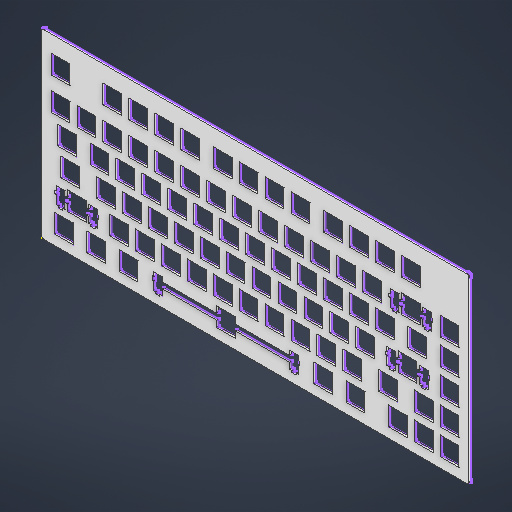
# Autodesk Inventor part: Keyboard_Plate
Saved by Autodesk Inventor 2026.1 (Build 301233000, 233)
## iProperties
Created: 2025-11-09
Part Number: Keyboard_Plate
Material: Generic
Document SubType Name: Modeling
Designer: avani
Density: 1 g/cm^3
Appearance: Default
Autodesk Inventor part; units mm, degrees
ref_plane "YZ Plane" through (0, 0, 0) normal (1, 0, 0) x (0, 1, 0)
ref_plane "XZ Plane" through (0, 0, 0) normal (0, 1, 0) x (-1, 0, 0)
ref_plane "XY Plane" through (0, 0, 0) normal (0, 0, 1) x (1, 0, 0)
sketch "Sketch1" plane through (0, 0, 0) normal (0, 0, 1) x (1, 0, 0)
  point P0 (0, 0)
sketch3d "3D 0"
sketch "Sketch2" plane through (0, 0, 0) normal (0, 0, 1) x (1, 0, 0)
  line L0 (2.096, 0.2549) -> (1.9389, 0.2604) projected
  line L1 (1.9389, 0.2604) -> (1.7818, 0.2797) projected
  line L2 (1.7818, 0.2797) -> (1.6288, 0.3087) projected
  line L3 (0.9192, 0.6367) -> (0.7965, 0.7331) projected
  line L4 (1.0501, 0.5498) -> (0.9192, 0.6367) projected
  line L5 (1.1879, 0.4727) -> (1.0501, 0.5498) projected
  line L6 (1.3298, 0.4065) -> (1.1879, 0.4727) projected
  line L7 (1.4759, 0.3528) -> (1.3298, 0.4065) projected
  line L8 (1.6288, 0.3087) -> (1.4759, 0.3528) projected
  line L9 (0.6808, 0.8406) -> (0.5746, 0.955) projected
  line L10 (0.5746, 0.955) -> (0.4768, 1.0776) projected
  line L11 (0.4768, 1.0776) -> (0.39, 1.2099) projected
  line L12 (0.39, 1.2099) -> (0.3128, 1.3463) projected
  line L13 (0.3128, 1.3463) -> (0.248, 1.4897) projected
  line L14 (0.7965, 0.7331) -> (0.6808, 0.8406) projected
  line L15 (0.248, 1.4897) -> (0.1929, 1.6357) projected
  line L16 (0.1929, 1.6357) -> (0.1502, 1.7873) projected
  line L17 (0.1502, 1.7873) -> (0.1199, 1.9417) projected
  line L18 (0.102, 2.0974) -> (0.0951, 2.2545) projected
  line L19 (0.1199, 1.9417) -> (0.102, 2.0974) projected
  line L20 (0.0951, 2.2545) -> (0.0951, 131.607) projected
  line L21 (0.0951, 131.607) -> (0.102, 131.764) projected
  line L22 (0.102, 131.764) -> (0.1199, 131.921) projected
  line L23 (0.5746, 132.906) -> (0.6808, 133.022) projected
  line L24 (0.6808, 133.022) -> (0.7965, 133.128) projected
  line L25 (0.7965, 133.128) -> (0.9192, 133.226) projected
  line L26 (0.9192, 133.226) -> (1.0501, 133.313) projected
  line L27 (1.0501, 133.313) -> (1.1879, 133.39) projected
  line L28 (1.1879, 133.39) -> (1.3298, 133.455) projected
  line L29 (0.1199, 131.921) -> (0.1502, 132.074) projected
  line L30 (0.1502, 132.074) -> (0.1929, 132.227) projected
  line L31 (0.1929, 132.227) -> (0.248, 132.373) projected
  line L32 (0.3128, 132.515) -> (0.39, 132.653) projected
  line L33 (0.39, 132.653) -> (0.4768, 132.784) projected
  line L34 (0.4768, 132.784) -> (0.5746, 132.906) projected
  line L35 (0.248, 132.373) -> (0.3128, 132.515) projected
  line L36 (1.3298, 133.455) -> (1.4759, 133.51) projected
  line L37 (1.4759, 133.51) -> (1.6288, 133.552) projected
  line L38 (1.6288, 133.552) -> (1.7818, 133.583) projected
  line L39 (1.7818, 133.583) -> (1.9389, 133.601) projected
  line L40 (1.9389, 133.601) -> (2.096, 133.608) projected
  line L41 (261.727, 40.4206) -> (261.727, 26.6209) projected
  line L42 (247.927, 26.6209) -> (247.927, 40.4206) projected
  line L43 (247.927, 40.4206) -> (261.727, 40.4206) projected
  line L44 (253.938, 45.8996) -> (255.662, 45.8996) projected
  line L45 (255.662, 45.8996) -> (255.662, 44.7008) projected
  line L46 (258.764, 44.7008) -> (258.764, 45.8996) projected
  line L47 (253.112, 52.1698) -> (253.938, 52.1698) projected
  line L48 (253.938, 52.1698) -> (253.938, 45.8996) projected
  line L49 (255.662, 44.7008) -> (258.764, 44.7008) projected
  line L50 (262.213, 59.4706) -> (262.213, 54.7702) projected
  line L51 (262.213, 54.7702) -> (260.488, 54.7702) projected
  line L52 (253.938, 54.7702) -> (253.112, 54.7702) projected
  line L53 (253.112, 54.7702) -> (253.112, 52.1698) projected
  line L54 (260.488, 54.7702) -> (260.488, 58.0002) projected
  line L55 (260.488, 58.0002) -> (253.938, 58.0002) projected
  line L56 (253.938, 58.0002) -> (253.938, 54.7702) projected
  line L57 (245.546, 78.5206) -> (259.345, 78.5206) projected
  line L58 (259.345, 78.5206) -> (259.345, 64.721) projected
  line L59 (259.345, 64.721) -> (245.546, 64.721) projected
  line L60 (245.546, 64.721) -> (245.546, 78.5206) projected
  line L61 (256.321, 90.2698) -> (256.321, 83.9996) projected
  line L62 (256.321, 83.9996) -> (258.046, 83.9996) projected
  line L63 (258.046, 83.9996) -> (258.046, 82.8008) projected
  line L64 (261.145, 83.9996) -> (262.871, 83.9996) projected
  line L65 (258.046, 82.8008) -> (261.145, 82.8008) projected
  line L66 (261.145, 82.8008) -> (261.145, 83.9996) projected
  line L67 (264.596, 107.582) -> (264.596, 121.382) projected
  line L68 (259.345, 121.382) -> (259.345, 107.582) projected
  line L69 (259.345, 107.582) -> (245.546, 107.582) projected
  line L70 (245.546, 107.582) -> (245.546, 121.382) projected
  line L71 (245.546, 121.382) -> (259.345, 121.382) projected
  line L72 (264.596, 92.8702) -> (262.871, 92.8702) projected
  line L73 (262.871, 92.8702) -> (262.871, 96.1002) projected
  line L74 (262.871, 96.1002) -> (256.321, 96.1002) projected
  line L75 (255.495, 90.2698) -> (256.321, 90.2698) projected
  line L76 (255.495, 92.8702) -> (255.495, 90.2698) projected
  line L77 (256.321, 92.8702) -> (255.495, 92.8702) projected
  line L78 (256.321, 96.1002) -> (256.321, 92.8702) projected
  line L79 (264.596, 97.5706) -> (264.596, 92.8702) projected
  line L80 (280.121, 92.8702) -> (278.395, 92.8702) projected
  line L81 (278.395, 92.8702) -> (278.395, 97.5706) projected
  line L82 (278.395, 97.5706) -> (264.596, 97.5706) projected
  line L83 (278.395, 107.582) -> (264.596, 107.582) projected
  line L84 (278.395, 121.382) -> (278.395, 107.582) projected
  line L85 (264.596, 121.382) -> (278.395, 121.382) projected
  line L86 (280.121, 96.1002) -> (280.121, 92.8702) projected
  line L87 (255.071, 21.3706) -> (268.87, 21.3706) projected
  line L88 (268.87, 21.3706) -> (268.87, 7.5709) projected
  line L89 (268.87, 7.5709) -> (255.071, 7.5709) projected
  line L90 (261.727, 26.6209) -> (247.927, 26.6209) projected
  line L91 (255.071, 7.5709) -> (255.071, 21.3706) projected
  line L92 (260.488, 45.8996) -> (260.488, 50.37) projected
  line L93 (258.764, 45.8996) -> (260.488, 45.8996) projected
  line L94 (262.213, 50.37) -> (262.213, 45.671) projected
  line L95 (260.488, 50.37) -> (262.213, 50.37) projected
  line L96 (262.213, 45.671) -> (276.014, 45.671) projected
  line L97 (283.158, 64.721) -> (269.357, 64.721) projected
  line L98 (276.014, 59.4706) -> (262.213, 59.4706) projected
  line L99 (283.158, 78.5206) -> (283.158, 64.721) projected
  line L100 (269.357, 64.721) -> (269.357, 78.5206) projected
  line L101 (269.357, 78.5206) -> (283.158, 78.5206) projected
  line L102 (264.596, 83.771) -> (278.395, 83.771) projected
  line L103 (278.395, 83.771) -> (278.395, 88.47) projected
  line L104 (262.871, 88.47) -> (264.596, 88.47) projected
  line L105 (262.871, 83.9996) -> (262.871, 88.47) projected
  line L106 (264.596, 88.47) -> (264.596, 83.771) projected
  line L107 (279.463, 44.7008) -> (282.564, 44.7008) projected
  line L108 (284.288, 45.8996) -> (284.288, 52.1698) projected
  line L109 (284.288, 52.1698) -> (285.113, 52.1698) projected
  line L110 (285.113, 52.1698) -> (285.113, 54.7702) projected
  line L111 (285.113, 54.7702) -> (284.288, 54.7702) projected
  line L112 (282.564, 45.8996) -> (284.288, 45.8996) projected
  line L113 (282.564, 44.7008) -> (282.564, 45.8996) projected
  line L114 (284.945, 82.8008) -> (284.945, 83.9996) projected
  line L115 (284.945, 83.9996) -> (286.67, 83.9996) projected
  line L116 (281.846, 83.9996) -> (281.846, 82.8008) projected
  line L117 (286.67, 83.9996) -> (286.67, 90.2698) projected
  line L118 (280.121, 83.9996) -> (281.846, 83.9996) projected
  line L119 (280.121, 88.47) -> (280.121, 83.9996) projected
  line L120 (278.395, 88.47) -> (280.121, 88.47) projected
  line L121 (281.846, 82.8008) -> (284.945, 82.8008) projected
  line L122 (286.67, 90.2698) -> (287.496, 90.2698) projected
  line L123 (287.496, 90.2698) -> (287.496, 92.8702) projected
  line L124 (287.496, 92.8702) -> (286.67, 92.8702) projected
  line L125 (286.67, 92.8702) -> (286.67, 96.1002) projected
  line L126 (286.67, 96.1002) -> (280.121, 96.1002) projected
  line L127 (274.121, 40.4206) -> (287.92, 40.4206) projected
  line L128 (287.92, 40.4206) -> (287.92, 26.6209) projected
  line L129 (287.92, 26.6209) -> (274.121, 26.6209) projected
  line L130 (274.121, 26.6209) -> (274.121, 40.4206) projected
  line L131 (277.738, 45.8996) -> (279.463, 45.8996) projected
  line L132 (277.738, 50.37) -> (277.738, 45.8996) projected
  line L133 (276.014, 45.671) -> (276.014, 50.37) projected
  line L134 (276.014, 50.37) -> (277.738, 50.37) projected
  line L135 (279.463, 45.8996) -> (279.463, 44.7008) projected
  line L136 (293.171, 97.5706) -> (306.97, 97.5706) projected
  line L137 (293.171, 83.771) -> (293.171, 97.5706) projected
  line L138 (306.97, 97.5706) -> (306.97, 83.771) projected
  line L139 (306.97, 83.771) -> (293.171, 83.771) projected
  line L140 (293.171, 59.4706) -> (306.97, 59.4706) projected
  line L141 (306.97, 59.4706) -> (306.97, 45.671) projected
  line L142 (306.97, 45.671) -> (293.171, 45.671) projected
  line L143 (293.171, 45.671) -> (293.171, 59.4706) projected
  line L144 (293.171, 78.5206) -> (306.97, 78.5206) projected
  line L145 (293.171, 64.721) -> (293.171, 78.5206) projected
  line L146 (306.97, 78.5206) -> (306.97, 64.721) projected
  line L147 (306.97, 64.721) -> (293.171, 64.721) projected
  line L148 (274.121, 21.3706) -> (287.92, 21.3706) projected
  line L149 (306.97, 21.3706) -> (306.97, 7.5709) projected
  line L150 (306.97, 7.5709) -> (293.171, 7.5709) projected
  line L151 (293.171, 7.5709) -> (293.171, 21.3706) projected
  line L152 (287.92, 21.3706) -> (287.92, 7.5709) projected
  line L153 (287.92, 7.5709) -> (274.121, 7.5709) projected
  line L154 (274.121, 7.5709) -> (274.121, 21.3706) projected
  line L155 (293.171, 21.3706) -> (306.97, 21.3706) projected
  line L156 (306.97, 26.6209) -> (293.171, 26.6209) projected
  line L157 (293.171, 26.6209) -> (293.171, 40.4206) projected
  line L158 (306.97, 40.4206) -> (306.97, 26.6209) projected
  line L159 (293.171, 40.4206) -> (306.97, 40.4206) projected
  line L160 (312.452, 133.601) -> (312.608, 133.583) projected
  line L161 (312.297, 133.608) -> (312.452, 133.601) projected
  line L162 (312.608, 133.583) -> (312.762, 133.552) projected
  line L163 (312.762, 133.552) -> (312.914, 133.51) projected
  line L164 (312.914, 133.51) -> (313.061, 133.455) projected
  line L165 (313.203, 133.39) -> (313.341, 133.313) projected
  line L166 (313.341, 133.313) -> (313.472, 133.226) projected
  line L167 (313.472, 133.226) -> (313.595, 133.128) projected
  line L168 (313.595, 133.128) -> (313.71, 133.022) projected
  line L169 (226.496, 107.582) -> (226.496, 121.382) projected
  line L170 (240.295, 107.582) -> (226.496, 107.582) projected
  line L171 (221.245, 121.382) -> (221.245, 107.582) projected
  line L172 (221.245, 107.582) -> (207.446, 107.582) projected
  line L173 (207.446, 107.582) -> (207.446, 121.382) projected
  line L174 (314.296, 131.607) -> (314.296, 2.2545) projected
  line L175 (2.096, 133.608) -> (312.297, 133.608) projected
  line L176 (312.297, 0.2549) -> (2.096, 0.2549) projected
  line L177 (226.496, 121.382) -> (240.295, 121.382) projected
  line L178 (313.71, 133.022) -> (313.817, 132.906) projected
  line L179 (313.061, 133.455) -> (313.203, 133.39) projected
  line L180 (207.446, 121.382) -> (221.245, 121.382) projected
  line L181 (183.632, 26.6209) -> (183.632, 40.4206) projected
  line L182 (178.383, 40.4206) -> (178.383, 26.6209) projected
  line L183 (178.383, 26.6209) -> (164.582, 26.6209) projected
  line L184 (164.582, 40.4206) -> (178.383, 40.4206) projected
  line L185 (164.582, 26.6209) -> (164.582, 40.4206) projected
  line L186 (187.908, 45.671) -> (174.107, 45.671) projected
  line L187 (187.908, 59.4706) -> (187.908, 45.671) projected
  line L188 (174.107, 59.4706) -> (187.908, 59.4706) projected
  line L189 (183.145, 64.721) -> (169.346, 64.721) projected
  line L190 (169.346, 78.5206) -> (183.145, 78.5206) projected
  line L191 (169.346, 64.721) -> (169.346, 78.5206) projected
  line L192 (174.107, 45.671) -> (174.107, 59.4706) projected
  line L193 (182.488, 12.2701) -> (182.488, 7.8011) projected
  line L194 (182.488, 7.8011) -> (184.213, 7.8011) projected
  line L195 (184.213, 7.8011) -> (184.213, 6.6008) projected
  line L196 (189.863, 16.6701) -> (189.038, 16.6701) projected
  line L197 (189.863, 14.0698) -> (189.863, 16.6701) projected
  line L198 (189.038, 14.0698) -> (189.863, 14.0698) projected
  line L199 (189.038, 7.8011) -> (189.038, 14.0698) projected
  line L200 (187.314, 7.8011) -> (189.038, 7.8011) projected
  line L201 (187.314, 6.6008) -> (187.314, 7.8011) projected
  line L202 (184.213, 6.6008) -> (187.314, 6.6008) projected
  line L203 (189.038, 19.9003) -> (182.488, 19.9003) projected
  line L204 (189.038, 16.6701) -> (189.038, 19.9003) projected
  line L205 (197.433, 26.6209) -> (183.632, 26.6209) projected
  line L206 (183.632, 40.4206) -> (197.433, 40.4206) projected
  line L207 (197.433, 40.4206) -> (197.433, 26.6209) projected
  line L208 (193.157, 45.671) -> (193.157, 59.4706) projected
  line L209 (206.958, 59.4706) -> (206.958, 45.671) projected
  line L210 (206.958, 45.671) -> (193.157, 45.671) projected
  line L211 (183.145, 78.5206) -> (183.145, 64.721) projected
  line L212 (193.157, 59.4706) -> (206.958, 59.4706) projected
  line L213 (202.195, 64.721) -> (188.396, 64.721) projected
  line L214 (188.396, 64.721) -> (188.396, 78.5206) projected
  line L215 (202.195, 78.5206) -> (202.195, 64.721) projected
  line L216 (211.72, 83.771) -> (197.921, 83.771) projected
  line L217 (211.72, 97.5706) -> (211.72, 83.771) projected
  line L218 (197.921, 97.5706) -> (211.72, 97.5706) projected
  line L219 (197.921, 83.771) -> (197.921, 97.5706) projected
  line L220 (192.67, 97.5706) -> (192.67, 83.771) projected
  line L221 (188.396, 78.5206) -> (202.195, 78.5206) projected
  line L222 (216.483, 40.4206) -> (216.483, 26.6209) projected
  line L223 (221.732, 26.6209) -> (221.732, 40.4206) projected
  line L224 (216.483, 26.6209) -> (202.682, 26.6209) projected
  line L225 (202.682, 26.6209) -> (202.682, 40.4206) projected
  line L226 (202.682, 40.4206) -> (216.483, 40.4206) projected
  line L227 (200.302, 21.3706) -> (214.102, 21.3706) projected
  line L228 (214.102, 21.3706) -> (214.102, 7.5709) projected
  line L229 (214.102, 7.5709) -> (200.302, 7.5709) projected
  line L230 (200.302, 7.5709) -> (200.302, 21.3706) projected
  line L231 (224.113, 21.3706) -> (237.914, 21.3706) projected
  line L232 (221.732, 40.4206) -> (235.533, 40.4206) projected
  line L233 (235.533, 40.4206) -> (235.533, 26.6209) projected
  line L234 (235.533, 26.6209) -> (221.732, 26.6209) projected
  line L235 (237.914, 21.3706) -> (237.914, 7.5709) projected
  line L236 (237.914, 7.5709) -> (224.113, 7.5709) projected
  line L237 (224.113, 7.5709) -> (224.113, 21.3706) projected
  line L238 (226.496, 78.5206) -> (240.295, 78.5206) projected
  line L239 (240.295, 78.5206) -> (240.295, 64.721) projected
  line L240 (226.496, 64.721) -> (226.496, 78.5206) projected
  line L241 (221.245, 64.721) -> (207.446, 64.721) projected
  line L242 (207.446, 78.5206) -> (221.245, 78.5206) projected
  line L243 (207.446, 64.721) -> (207.446, 78.5206) projected
  line L244 (221.245, 78.5206) -> (221.245, 64.721) projected
  line L245 (226.008, 45.671) -> (212.207, 45.671) projected
  line L246 (245.058, 45.671) -> (231.257, 45.671) projected
  line L247 (231.257, 45.671) -> (231.257, 59.4706) projected
  line L248 (231.257, 59.4706) -> (245.058, 59.4706) projected
  line L249 (245.058, 59.4706) -> (245.058, 45.671) projected
  line L250 (240.295, 64.721) -> (226.496, 64.721) projected
  line L251 (226.008, 59.4706) -> (226.008, 45.671) projected
  line L252 (212.207, 59.4706) -> (226.008, 59.4706) projected
  line L253 (212.207, 45.671) -> (212.207, 59.4706) projected
  line L254 (230.77, 83.771) -> (216.971, 83.771) projected
  line L255 (249.82, 83.771) -> (236.021, 83.771) projected
  line L256 (216.971, 97.5706) -> (230.77, 97.5706) projected
  line L257 (216.971, 83.771) -> (216.971, 97.5706) projected
  line L258 (230.77, 97.5706) -> (230.77, 83.771) projected
  line L259 (236.021, 83.771) -> (236.021, 97.5706) projected
  line L260 (249.82, 97.5706) -> (249.82, 83.771) projected
  line L261 (236.021, 97.5706) -> (249.82, 97.5706) projected
  line L262 (240.295, 121.382) -> (240.295, 107.582) projected
  line L263 (314.289, 131.764) -> (314.296, 131.607) projected
  line L264 (314.271, 131.921) -> (314.289, 131.764) projected
  line L265 (314.241, 132.074) -> (314.271, 131.921) projected
  line L266 (313.817, 132.906) -> (313.914, 132.784) projected
  line L267 (313.914, 132.784) -> (314.001, 132.653) projected
  line L268 (314.001, 132.653) -> (314.078, 132.515) projected
  line L269 (314.078, 132.515) -> (314.143, 132.373) projected
  line L270 (314.143, 132.373) -> (314.198, 132.227) projected
  line L271 (314.198, 132.227) -> (314.241, 132.074) projected
  line L272 (313.061, 0.4065) -> (312.914, 0.3528) projected
  line L273 (312.914, 0.3528) -> (312.762, 0.3087) projected
  line L274 (312.762, 0.3087) -> (312.608, 0.2797) projected
  line L275 (312.608, 0.2797) -> (312.452, 0.2604) projected
  line L276 (312.452, 0.2604) -> (312.297, 0.2549) projected
  line L277 (313.203, 0.4727) -> (313.061, 0.4065) projected
  line L278 (313.914, 1.0776) -> (313.817, 0.955) projected
  line L279 (313.817, 0.955) -> (313.71, 0.8406) projected
  line L280 (313.71, 0.8406) -> (313.595, 0.7331) projected
  line L281 (313.595, 0.7331) -> (313.472, 0.6367) projected
  line L282 (313.472, 0.6367) -> (313.341, 0.5498) projected
  line L283 (313.341, 0.5498) -> (313.203, 0.4727) projected
  line L284 (314.296, 2.2545) -> (314.289, 2.0974) projected
  line L285 (314.289, 2.0974) -> (314.271, 1.9417) projected
  line L286 (314.001, 1.2099) -> (313.914, 1.0776) projected
  line L287 (314.078, 1.3463) -> (314.001, 1.2099) projected
  line L288 (314.143, 1.4897) -> (314.078, 1.3463) projected
  line L289 (314.198, 1.6357) -> (314.143, 1.4897) projected
  line L290 (314.241, 1.7873) -> (314.198, 1.6357) projected
  line L291 (314.271, 1.9417) -> (314.241, 1.7873) projected
  line L292 (89.0379, 16.6701) -> (89.0379, 19.9003) projected
  line L293 (89.0379, 19.9003) -> (82.4879, 19.9003) projected
  line L294 (81.6638, 14.0698) -> (82.4879, 14.0698) projected
  line L295 (81.6638, 16.6701) -> (81.6638, 14.0698) projected
  line L296 (82.4879, 16.6701) -> (81.6638, 16.6701) projected
  line L297 (82.4879, 19.9003) -> (82.4879, 16.6701) projected
  line L298 (82.4879, 14.0698) -> (82.4879, 7.8011) projected
  line L299 (82.4879, 7.8011) -> (84.2133, 7.8011) projected
  line L300 (89.0379, 7.8011) -> (89.0379, 12.2701) projected
  line L301 (84.2133, 7.8011) -> (84.2133, 6.6008) projected
  line L302 (87.3139, 7.8011) -> (89.0379, 7.8011) projected
  line L303 (87.3139, 6.6008) -> (87.3139, 7.8011) projected
  line L304 (84.2133, 6.6008) -> (87.3139, 6.6008) projected
  line L305 (97.4203, 83.771) -> (83.6193, 83.771) projected
  line L306 (102.669, 83.771) -> (102.669, 97.5706) projected
  line L307 (97.4203, 97.5706) -> (97.4203, 83.771) projected
  line L308 (83.6193, 83.771) -> (83.6193, 97.5706) projected
  line L309 (83.6193, 97.5706) -> (97.4203, 97.5706) projected
  line L310 (83.1328, 40.4206) -> (83.1328, 26.6209) projected
  line L311 (102.183, 40.4206) -> (102.183, 26.6209) projected
  line L312 (102.183, 26.6209) -> (88.3818, 26.6209) projected
  line L313 (92.6578, 45.671) -> (78.8568, 45.671) projected
  line L314 (88.3818, 40.4206) -> (102.183, 40.4206) projected
  line L315 (78.8568, 45.671) -> (78.8568, 59.4706) projected
  line L316 (78.8568, 59.4706) -> (92.6578, 59.4706) projected
  line L317 (92.6578, 59.4706) -> (92.6578, 45.671) projected
  line L318 (97.9068, 45.671) -> (97.9068, 59.4706) projected
  line L319 (87.8953, 78.5206) -> (87.8953, 64.721) projected
  line L320 (87.8953, 64.721) -> (74.0943, 64.721) projected
  line L321 (74.0943, 78.5206) -> (87.8953, 78.5206) projected
  line L322 (74.0943, 64.721) -> (74.0943, 78.5206) projected
  line L323 (93.1443, 64.721) -> (93.1443, 78.5206) projected
  line L324 (64.5707, 97.5706) -> (78.3703, 97.5706) projected
  line L325 (78.3703, 97.5706) -> (78.3703, 83.771) projected
  line L326 (78.3703, 83.771) -> (64.5707, 83.771) projected
  line L327 (64.5707, 83.771) -> (64.5707, 97.5706) projected
  line L328 (64.5707, 107.582) -> (64.5707, 121.382) projected
  line L329 (64.5707, 121.382) -> (78.3703, 121.382) projected
  line L330 (78.3703, 107.582) -> (64.5707, 107.582) projected
  line L331 (78.3703, 121.382) -> (78.3703, 107.582) projected
  line L332 (83.6193, 121.382) -> (97.4203, 121.382) projected
  line L333 (97.4203, 107.582) -> (83.6193, 107.582) projected
  line L334 (83.6193, 107.582) -> (83.6193, 121.382) projected
  line L335 (83.1328, 26.6209) -> (69.3318, 26.6209) projected
  line L336 (88.3818, 26.6209) -> (88.3818, 40.4206) projected
  line L337 (69.3318, 40.4206) -> (83.1328, 40.4206) projected
  line L338 (69.3318, 26.6209) -> (69.3318, 40.4206) projected
  line L339 (64.0828, 40.4206) -> (64.0828, 26.6209) projected
  line L340 (57.4269, 21.3706) -> (71.2265, 21.3706) projected
  line L341 (50.2818, 40.4206) -> (64.0828, 40.4206) projected
  line L342 (50.2818, 26.6209) -> (50.2818, 40.4206) projected
  line L343 (64.0828, 26.6209) -> (50.2818, 26.6209) projected
  line L344 (71.2265, 21.3706) -> (71.2265, 7.5709) projected
  line L345 (71.2265, 7.5709) -> (57.4269, 7.5709) projected
  line L346 (57.4269, 7.5709) -> (57.4269, 21.3706) projected
  line L347 (40.7568, 59.4706) -> (54.5578, 59.4706) projected
  line L348 (54.5578, 59.4706) -> (54.5578, 45.671) projected
  line L349 (54.5578, 45.671) -> (40.7568, 45.671) projected
  line L350 (40.7568, 45.671) -> (40.7568, 59.4706) projected
  line L351 (59.8068, 59.4706) -> (73.6078, 59.4706) projected
  line L352 (55.0443, 78.5206) -> (68.8453, 78.5206) projected
  line L353 (68.8453, 78.5206) -> (68.8453, 64.721) projected
  line L354 (68.8453, 64.721) -> (55.0443, 64.721) projected
  line L355 (59.8068, 45.671) -> (59.8068, 59.4706) projected
  line L356 (73.6078, 59.4706) -> (73.6078, 45.671) projected
  line L357 (73.6078, 45.671) -> (59.8068, 45.671) projected
  line L358 (45.5207, 97.5706) -> (59.3189, 97.5706) projected
  line L359 (59.3189, 107.582) -> (45.5207, 107.582) projected
  line L360 (45.5207, 121.382) -> (59.3189, 121.382) projected
  line L361 (59.3189, 121.382) -> (59.3189, 107.582) projected
  line L362 (59.3189, 83.771) -> (45.5207, 83.771) projected
  line L363 (45.5207, 83.771) -> (45.5207, 97.5706) projected
  line L364 (59.3189, 97.5706) -> (59.3189, 83.771) projected
  line L365 (55.0443, 64.721) -> (55.0443, 78.5206) projected
  line L366 (49.7939, 64.721) -> (35.9957, 64.721) projected
  line L367 (35.9957, 78.5206) -> (49.7939, 78.5206) projected
  line L368 (35.9957, 64.721) -> (35.9957, 78.5206) projected
  line L369 (49.7939, 78.5206) -> (49.7939, 64.721) projected
  line L370 (40.2703, 83.771) -> (26.4708, 83.771) projected
  line L371 (26.4708, 83.771) -> (26.4708, 97.5706) projected
  line L372 (26.4708, 97.5706) -> (40.2703, 97.5706) projected
  line L373 (40.2703, 97.5706) -> (40.2703, 83.771) projected
  line L374 (45.5207, 107.582) -> (45.5207, 121.382) projected
  line L375 (7.4207, 97.5706) -> (21.2204, 97.5706) projected
  line L376 (21.2204, 97.5706) -> (21.2204, 83.771) projected
  line L377 (21.2204, 83.771) -> (7.4207, 83.771) projected
  line L378 (7.4207, 83.771) -> (7.4207, 97.5706) projected
  line L379 (21.2204, 121.382) -> (21.2204, 107.582) projected
  line L380 (21.2204, 107.582) -> (7.4207, 107.582) projected
  line L381 (7.4207, 107.582) -> (7.4207, 121.382) projected
  line L382 (7.4207, 121.382) -> (21.2204, 121.382) projected
  line L383 (25.9829, 64.721) -> (12.1819, 64.721) projected
  line L384 (25.9829, 78.5206) -> (25.9829, 64.721) projected
  line L385 (12.1819, 78.5206) -> (25.9829, 78.5206) projected
  line L386 (12.1819, 64.721) -> (12.1819, 78.5206) projected
  line L387 (42.2257, 33.1198) -> (42.2257, 35.7202) projected
  line L388 (42.2257, 35.7202) -> (41.4016, 35.7202) projected
  line L389 (41.4016, 35.7202) -> (41.4016, 38.9502) projected
  line L390 (41.4016, 38.9502) -> (34.852, 38.9502) projected
  line L391 (34.852, 35.7202) -> (33.1266, 35.7202) projected
  line L392 (34.852, 38.9502) -> (34.852, 35.7202) projected
  line L393 (33.1266, 35.7202) -> (33.1266, 40.4206) projected
  line L394 (34.852, 31.3201) -> (34.852, 26.8497) projected
  line L395 (34.852, 26.8497) -> (36.576, 26.8497) projected
  line L396 (36.576, 26.8497) -> (36.576, 25.6508) projected
  line L397 (36.576, 25.6508) -> (39.6766, 25.6508) projected
  line L398 (39.6766, 25.6508) -> (39.6766, 26.8497) projected
  line L399 (39.6766, 26.8497) -> (41.4016, 26.8497) projected
  line L400 (41.4016, 26.8497) -> (41.4016, 33.1198) projected
  line L401 (41.4016, 33.1198) -> (42.2257, 33.1198) projected
  line L402 (33.1266, 40.4206) -> (19.327, 40.4206) projected
  line L403 (28.3641, 59.4706) -> (28.3641, 45.671) projected
  line L404 (14.5631, 59.4706) -> (28.3641, 59.4706) projected
  line L405 (14.5631, 45.671) -> (14.5631, 59.4706) projected
  line L406 (28.3641, 45.671) -> (14.5631, 45.671) projected
  line L407 (15.8764, 26.8497) -> (17.6017, 26.8497) projected
  line L408 (17.6017, 26.8497) -> (17.6017, 31.3201) projected
  line L409 (17.6017, 31.3201) -> (19.327, 31.3201) projected
  line L410 (19.327, 40.4206) -> (19.327, 35.7202) projected
  line L411 (19.327, 35.7202) -> (17.6017, 35.7202) projected
  line L412 (10.2264, 33.1198) -> (11.0519, 33.1198) projected
  line L413 (10.2264, 35.7202) -> (10.2264, 33.1198) projected
  line L414 (17.6017, 35.7202) -> (17.6017, 38.9502) projected
  line L415 (17.6017, 38.9502) -> (11.0519, 38.9502) projected
  line L416 (11.0519, 38.9502) -> (11.0519, 35.7202) projected
  line L417 (11.0519, 35.7202) -> (10.2264, 35.7202) projected
  line L418 (33.6131, 21.3706) -> (47.414, 21.3706) projected
  line L419 (47.414, 21.3706) -> (47.414, 7.5709) projected
  line L420 (47.414, 7.5709) -> (33.6131, 7.5709) projected
  line L421 (33.6131, 7.5709) -> (33.6131, 21.3706) projected
  line L422 (19.327, 26.6209) -> (33.1266, 26.6209) projected
  line L423 (33.1266, 26.6209) -> (33.1266, 31.3201) projected
  line L424 (33.1266, 31.3201) -> (34.852, 31.3201) projected
  line L425 (19.327, 31.3201) -> (19.327, 26.6209) projected
  line L426 (9.802, 21.3706) -> (23.6016, 21.3706) projected
  line L427 (23.6016, 21.3706) -> (23.6016, 7.5709) projected
  line L428 (23.6016, 7.5709) -> (9.802, 7.5709) projected
  line L429 (9.802, 7.5709) -> (9.802, 21.3706) projected
  line L430 (11.0519, 33.1198) -> (11.0519, 26.8497) projected
  line L431 (11.0519, 26.8497) -> (12.7772, 26.8497) projected
  line L432 (12.7772, 26.8497) -> (12.7772, 25.6508) projected
  line L433 (15.8764, 25.6508) -> (15.8764, 26.8497) projected
  line L434 (12.7772, 25.6508) -> (15.8764, 25.6508) projected
  line L435 (284.288, 54.7702) -> (284.288, 58.0002) projected
  line L436 (284.288, 58.0002) -> (277.738, 58.0002) projected
  line L437 (277.738, 54.7702) -> (276.014, 54.7702) projected
  line L438 (277.738, 58.0002) -> (277.738, 54.7702) projected
  line L439 (276.014, 54.7702) -> (276.014, 59.4706) projected
  line L440 (128.863, 21.3706) -> (128.863, 16.6701) projected
  line L441 (128.863, 12.2701) -> (128.863, 7.5709) projected
  line L442 (126.482, 40.4206) -> (140.283, 40.4206) projected
  line L443 (140.283, 40.4206) -> (140.283, 26.6209) projected
  line L444 (140.283, 26.6209) -> (126.482, 26.6209) projected
  line L445 (142.664, 21.3706) -> (128.863, 21.3706) projected
  line L446 (142.664, 16.6701) -> (142.664, 21.3706) projected
  line L447 (128.863, 7.5709) -> (142.664, 7.5709) projected
  line L448 (111.708, 45.671) -> (97.9068, 45.671) projected
  line L449 (111.708, 59.4706) -> (111.708, 45.671) projected
  line L450 (97.9068, 59.4706) -> (111.708, 59.4706) projected
  line L451 (106.945, 64.721) -> (93.1443, 64.721) projected
  line L452 (93.1443, 78.5206) -> (106.945, 78.5206) projected
  line L453 (106.945, 78.5206) -> (106.945, 64.721) projected
  line L454 (116.47, 107.582) -> (102.669, 107.582) projected
  line L455 (116.47, 121.382) -> (116.47, 107.582) projected
  line L456 (102.669, 121.382) -> (116.47, 121.382) projected
  line L457 (102.669, 107.582) -> (102.669, 121.382) projected
  line L458 (97.4203, 121.382) -> (97.4203, 107.582) projected
  line L459 (116.47, 83.771) -> (102.669, 83.771) projected
  line L460 (102.669, 97.5706) -> (116.47, 97.5706) projected
  line L461 (116.47, 97.5706) -> (116.47, 83.771) projected
  line L462 (131.244, 64.721) -> (131.244, 78.5206) projected
  line L463 (125.994, 78.5206) -> (125.994, 64.721) projected
  line L464 (125.994, 64.721) -> (112.194, 64.721) projected
  line L465 (112.194, 78.5206) -> (125.994, 78.5206) projected
  line L466 (112.194, 64.721) -> (112.194, 78.5206) projected
  line L467 (135.52, 83.771) -> (121.721, 83.771) projected
  line L468 (135.52, 97.5706) -> (135.52, 83.771) projected
  line L469 (121.721, 83.771) -> (121.721, 97.5706) projected
  line L470 (121.721, 97.5706) -> (135.52, 97.5706) projected
  line L471 (128.863, 16.6701) -> (89.0379, 16.6701) projected
  line L472 (89.0379, 12.2701) -> (128.863, 12.2701) projected
  line L473 (126.482, 26.6209) -> (126.482, 40.4206) projected
  line L474 (121.233, 40.4206) -> (121.233, 26.6209) projected
  line L475 (121.233, 26.6209) -> (107.432, 26.6209) projected
  line L476 (107.432, 40.4206) -> (121.233, 40.4206) projected
  line L477 (107.432, 26.6209) -> (107.432, 40.4206) projected
  line L478 (116.957, 59.4706) -> (130.758, 59.4706) projected
  line L479 (130.758, 59.4706) -> (130.758, 45.671) projected
  line L480 (130.758, 45.671) -> (116.957, 45.671) projected
  line L481 (116.957, 45.671) -> (116.957, 59.4706) projected
  line L482 (136.007, 59.4706) -> (149.808, 59.4706) projected
  line L483 (131.244, 78.5206) -> (145.045, 78.5206) projected
  line L484 (145.045, 78.5206) -> (145.045, 64.721) projected
  line L485 (145.045, 64.721) -> (131.244, 64.721) projected
  line L486 (136.007, 45.671) -> (136.007, 59.4706) projected
  line L487 (149.808, 45.671) -> (136.007, 45.671) projected
  line L488 (149.808, 59.4706) -> (149.808, 45.671) projected
  line L489 (142.664, 7.5709) -> (142.664, 12.2701) projected
  line L490 (145.532, 40.4206) -> (159.333, 40.4206) projected
  line L491 (159.333, 40.4206) -> (159.333, 26.6209) projected
  line L492 (145.532, 26.6209) -> (145.532, 40.4206) projected
  line L493 (159.333, 26.6209) -> (145.532, 26.6209) projected
  line L494 (182.488, 19.9003) -> (182.488, 16.6701) projected
  line L495 (182.488, 16.6701) -> (142.664, 16.6701) projected
  line L496 (142.664, 12.2701) -> (182.488, 12.2701) projected
  line L497 (168.858, 45.671) -> (155.057, 45.671) projected
  line L498 (168.858, 59.4706) -> (168.858, 45.671) projected
  line L499 (155.057, 59.4706) -> (168.858, 59.4706) projected
  line L500 (155.057, 45.671) -> (155.057, 59.4706) projected
  line L501 (150.296, 78.5206) -> (164.095, 78.5206) projected
  line L502 (173.62, 83.771) -> (159.821, 83.771) projected
  line L503 (150.296, 64.721) -> (150.296, 78.5206) projected
  line L504 (164.095, 64.721) -> (150.296, 64.721) projected
  line L505 (164.095, 78.5206) -> (164.095, 64.721) projected
  line L506 (159.333, 107.582) -> (145.532, 107.582) projected
  line L507 (159.333, 121.382) -> (159.333, 107.582) projected
  line L508 (145.532, 121.382) -> (159.333, 121.382) projected
  line L509 (145.532, 107.582) -> (145.532, 121.382) projected
  line L510 (140.283, 121.382) -> (140.283, 107.582) projected
  line L511 (140.283, 107.582) -> (126.482, 107.582) projected
  line L512 (126.482, 121.382) -> (140.283, 121.382) projected
  line L513 (126.482, 107.582) -> (126.482, 121.382) projected
  line L514 (159.821, 97.5706) -> (173.62, 97.5706) projected
  line L515 (173.62, 97.5706) -> (173.62, 83.771) projected
  line L516 (154.57, 83.771) -> (140.771, 83.771) projected
  line L517 (159.821, 83.771) -> (159.821, 97.5706) projected
  line L518 (154.57, 97.5706) -> (154.57, 83.771) projected
  line L519 (140.771, 83.771) -> (140.771, 97.5706) projected
  line L520 (140.771, 97.5706) -> (154.57, 97.5706) projected
  line L521 (197.433, 107.582) -> (183.632, 107.582) projected
  line L522 (197.433, 121.382) -> (197.433, 107.582) projected
  line L523 (183.632, 121.382) -> (197.433, 121.382) projected
  line L524 (183.632, 107.582) -> (183.632, 121.382) projected
  line L525 (178.383, 121.382) -> (178.383, 107.582) projected
  line L526 (178.383, 107.582) -> (164.582, 107.582) projected
  line L527 (164.582, 121.382) -> (178.383, 121.382) projected
  line L528 (164.582, 107.582) -> (164.582, 121.382) projected
  line L529 (192.67, 83.771) -> (178.871, 83.771) projected
  line L530 (178.871, 83.771) -> (178.871, 97.5706) projected
  line L531 (178.871, 97.5706) -> (192.67, 97.5706) projected
  point P0 (0, 0)
  point P1 (0, 0)
extrude "Extrusion1" add sketch "Sketch2" along normal blind 1.5
body "Solid1"
